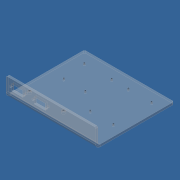
# Autodesk Inventor part: P1704_009
Saved by Autodesk Inventor 2015 SP2 (Build 190223200, 223)
## iProperties
Created: 2018-05-15
Part Number: P1704_009
Project: Manette arcade
Material: Plastique PMMA
Description: Plaque
Document SubType Name: Tôlerie
Designer: Alexandre.PICOTTE
Authority: 167x160x4
Sheet Metal Rule: Par défaut
Appearance: Transparent - Clair
Density: 1.188 g/cm^3
Flat Pattern Width: 16 cm
Flat Pattern Length: 16.7048 cm
Flat Pattern Area: 267.276 cm^2
Sheet Metal Width: 160.000 mm
Sheet Metal Length: 167.048 mm
Sheet Metal Area: 26727.646 mm^2
Mass: 124.568 g
Surface Area: 561.497 cm^2
Volume: 104.855 cm^3
Material number: ---
Author: Alexandre.PICOTTE
Autodesk Inventor part; units mm, degrees
ref_plane "Plan YZ" through (0, 0, 0) normal (1, 0, 0) x (0, 1, 0)
ref_plane "Plan XZ" through (0, 0, 0) normal (0, 1, 0) x (-1, 0, 0)
ref_plane "Plan XY" through (0, 0, 0) normal (0, 0, 1) x (1, 0, 0)
sketch "Esquisse1" plane through (0, 0, 0) normal (0, 0, 1) x (1, 0, 0)
  line L0 (-78, 70) -> (78, 70)
  line L1 (80, 68) -> (80, -68)
  line L2 (78, -70) -> (-78, -70)
  line L3 (-80, -68) -> (-80, 68)
  line L4 (-112, 0) -> (112, 0) construction
  line L5 (0, -98) -> (0, 98) construction
  line L6 (-80, 68) -> (-80, 70)
  line L7 (-80, 70) -> (-78, 70)
  line L8 (80, 68) -> (80, 70)
  line L9 (78, 70) -> (80, 70)
  line L10 (-78, -70) -> (-80, -70)
  line L11 (-80, -70) -> (-80, -68)
  line L12 (78, -70) -> (80, -70)
  line L13 (80, -70) -> (80, -68)
  point P0 (0, 0)
  dimension "d0" = 160
  dimension "d1" = 140
  constraints: 24 end point, 8 point on line, 5 perpendicular, 2 collinear, 2 horizontal, 2 parallel, 1 vertical, 2 other
  measures "d0" distance of L6.end L8.end
  measures "d1" distance of L10.end L6.end
extrude "Extrusion1" add sketch "Esquisse1" along normal blind 4
sketch "Esquisse5" plane through (0, 0, 4) normal (0, 0, 1) x (1, 0, 0)
  line L0 (18.6, 50) -> (60, 50) construction
  line L1 (60, 50) -> (60, -18.2) construction
  line L2 (60, -18.2) -> (18.6, -18.2) construction
  line L3 (18.6, -18.2) -> (18.6, 50) construction
  line L4 (80, -70.465) -> (80, 70)
  line L5 (80, 70) -> (-80, 70)
  line L6 (80, 70) -> (-80, 70) projected
  line L7 (80, -70) -> (80, 70) projected
  point P0 (0, 0)
  point P1 (0, 0)
  point P2 (78, 70)
  point P3 (-78, 70)
  point P4 (80, -68)
  point P5 (80, 68)
  dimension "d12" = 41.4
  dimension "d13" = 68.2
  dimension "d14" = 20
  dimension "d15" = 20
  constraints: 12 end point, 4 coincident, 2 collinear, 2 parallel, 1 horizontal, 1 perpendicular
  measures "d12" distance of L0.start L0.end
  measures "d13" distance of L2.end L0.start
  measures "d14" distance between parallel lines of L4 L1
  measures "d15" distance between parallel lines of L5 L0
hole "Perçage1" at (18.6, 50, 4) at (60, 50, 4) at (18.6, -18.2, 4) at (60, -18.2, 4) direction (0, 0, -1) diameter 2.459 end through all thread size "M3x0.5" class "6H" standard "ISO M"
sketch "Esquisse6" plane through (0, 0, 4) normal (0, 0, 1) x (1, 0, 0)
  line L0 (-60, 50) -> (-11.3, 50) construction
  line L1 (-11.3, 50) -> (-11.3, 8.1) construction
  line L2 (-11.3, 8.1) -> (-60, 8.1) construction
  line L3 (-60, 8.1) -> (-60, 50) construction
  line L4 (-35.65, 66.5768) -> (-35.65, 16.8329)
  line L5 (-80, 70) -> (-80, -63.3699)
  line L6 (-80, 70) -> (-80, -70) construction
  line L7 (80, 70) -> (-80, 70) projected
  circle A0 centre (18.6, 50) radius 1.2295 construction
  point P0 (0, 0)
  point P1 (0, 0)
  point P2 (-54.9, 8.1)
  point P3 (-16.4, 8.1)
  point P4 (-80, 68)
  point P5 (-80, -68)
  point P6 (78, 70)
  point P7 (-78, 70)
  dimension "d23" = 41.9
  dimension "d24" = 38.5
  dimension "d25" = 48.7
  dimension "d26" = 48.7
  dimension "d27" = 20
  constraints: 13 end point, 3 coincident, 3 point on line, 2 parallel, 1 collinear, 1 horizontal, 1 perpendicular, 1 symmetric about line, 1 vertical, 2 other
  measures "d23" distance of L2.end L0.start
  measures "d24" distance of point (-16.4, 8.1) point (-54.9, 8.1)
  measures "d25" diameter of L1 L4
  measures "d26" distance of L0.start L0.end
  measures "d27" distance between parallel lines of L5 L3
hole "Perçage2" at (-54.9, 8.1, 4) at (-16.4, 8.1, 4) at (-60, 50, 4) at (-11.3, 50, 4) direction (0, 0, -1) diameter 2.459 end through all thread size "M3x0.5" class "6H" standard "ISO M"
sketch "Esquisse10" plane through (80, -66, 0) normal (0, -1, 0) x (1, 0, 0)
  line L0 (-160, 0) -> (0, 0)
  line L1 (0, 0) -> (0, 34)
  line L2 (0, 34) -> (-160, 34)
  line L3 (-160, 34) -> (-160, 0)
  constraints: 6 end point, 1 horizontal, 1 perpendicular, 1 vertical
edge flange "Bord tombé2" height 34 angle 90 thickness 4 bend radius 4 thickness toward (0, -1, 0) relief tear relief width 4 relief depth 2 edges at (0, -70, 4) wall of the first edge with corners at (-80, -66, 0) (80, -66, 0) (80, -66, 34) (-80, -66, 34)
bend "Pli3"
corner "Coin2"
chamfer "Chanfrein1" distance 2 angle 45 4 edges at (-80, -68, 34) (80, -68, 34) (80, 70, 2) (-80, 70, 2)
sketch "Esquisse13" plane through (0, 0, 0) normal (0, 0, -1) x (-1, 0, 0)
  line L0 (35.65, 25.8994) -> (35.65, -17.0856) construction
  line L1 (80, -70) -> (-80, -70) construction
  line L2 (80, 68) -> (80, -62) construction
  line L3 (151.9558, 0) -> (-118.6593, 0) construction
  line L4 (80, -62) -> (-80, -62) projected
  point P0 (0, 0)
  point P1 (0, 0)
  point P2 (0, 0)
  point P3 (66.05, -42)
  point P4 (5.25, -42)
  point P5 (16.4, 8.1)
  dimension "d102" = 38.5
  dimension "d107" = 60.8
  dimension "d115" = 20
  constraints: 2 end point, 1 horizontal alignment, 1 symmetric about line
  measures "d102" diameter of point (16.4, 8.1) L0
  measures "d107" distance of point (5.25, -42) point (66.05, -42)
  measures "d115" distance from line of L4 point (66.05, -42)
hole "Perçage4" at (-5.25, -42, 0) at (-66.05, -42, 0) direction (0, 0, 1) diameter 3.4 end through all counterbore diameter 6.5 counterbore depth 2.8
sketch "Esquisse12" plane through (-80, -70, 8) normal (0, -1, 0) x (1, 0, 0)
  line L0 (10, 18.5) -> (30, 18.5)
  line L1 (30, 18.5) -> (30, 7.5)
  line L2 (30, 7.5) -> (10, 7.5)
  line L3 (10, 7.5) -> (10, 18.5)
  line L4 (50, 18.5) -> (70, 18.5)
  line L5 (70, 18.5) -> (70, 7.5)
  line L6 (70, 7.5) -> (50, 7.5)
  line L7 (50, 7.5) -> (50, 18.5)
  line L8 (2, 26) -> (158, 26)
  line L9 (-10.9148, 13) -> (171.3992, 13)
  line L10 (20, 22.4004) -> (20, 5.8983)
  circle A0 centre (7.503, 13) radius 1.7
  circle A1 centre (32.497, 13) radius 1.7
  circle A2 centre (47.503, 13) radius 1.7
  circle A3 centre (72.497, 13) radius 1.7
  line L11 (60, 25.3782) -> (60, 6.6427)
  line L12 (0, -0.9203) -> (0, 29.0797)
  line L13 (40, 26) -> (40, -5.9495)
  line L14 (0, 0) -> (0, 24) projected
  line L15 (2, 26) -> (158, 26) projected
  point P0 (80, -8)
  point P1 (80, -2)
  dimension "d81" = 26
  dimension "d82" = 11
  dimension "d83" = 20
  dimension "d84" = 20
  dimension "d85" = 20
  dimension "d86" = 24.994
  dimension "d87" = 3.4
  dimension "d88" = 24.994
  dimension "d89" = 20
  dimension "d90" = 80
  constraints: 28 end point, 7 point on line, 4 centre point, 4 parallel, 3 collinear, 3 equal radius, 3 horizontal, 3 perpendicular, 1 vertical, 4 other
  measures "d81" diameter of L8 L9
  measures "d82" distance of L2.end L0.start
  measures "d83" diameter of L1 L10
  measures "d84" distance of L0.start L0.end
  measures "d85" diameter of L5 L11
  measures "d86" distance of A0.centre A1.centre
  measures "d87" diameter of A0
  measures "d88" distance of A3.centre A2.centre
  measures "d89" distance between parallel lines of L7 L1
  measures "d90" diameter of L12 L13
extrude "Extrusion4" cut sketch "Esquisse12" against normal through all
equation "\"d26\" = d25"
equation "\"d102\" = d24"
equation "\"d113\" = Epaisseur"
equation "\"d88\" = d86"
equation "\"d90\" = 0.5 * d91"
equation "\"d65\" = LargeurGrugeage"
equation "\"d66\" = ProfondeurGrugeage"
equation "\"d67\" = RestesMinimum"
equation "\"d68\" = RayonPli"
equation "\"d71\" = RayonPli"
equation "\"d72\" = TailleGrugeage"
equation "\"d73\" = TailleJeu"
equation "\"d74\" = TailleRayonJacobi"
equation "\"RayonPli\" = Epaisseur"
equation "\"LargeurGrugeage\" = Epaisseur"
equation "\"ProfondeurGrugeage\" = 0.5 * Epaisseur"
equation "\"TailleGrugeage\" = 4 * Epaisseur"
equation "\"RestesMinimum\" = 2 * Epaisseur"
equation "\"Rayondetransition\" = RayonPli"
equation "\"TailleRayonJacobi\" = Epaisseur"
equation "\"TailleJeu\" = Epaisseur"
equation "\"Epaisseur\" = 4"
equation "\"d91\" = 160"
